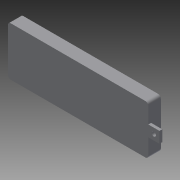
# Autodesk Inventor part: NodeMCU_holes
Saved by Autodesk Inventor 2014 SP1 (Build 180222100, 222)
## iProperties
Created: 2016-10-22
Part Number: NodeMCU_holes
Material: Generic
Document SubType Name: Modeling
Designer: danielsikar
Density: 1 g/cm^3
Appearance: Default
Author: danielsikar
Autodesk Inventor part; units mm, degrees
ref_plane "YZ Plane" through (0, 0, 0) normal (1, 0, 0) x (0, 1, 0)
ref_plane "XZ Plane" through (0, 0, 0) normal (0, 1, 0) x (-1, 0, 0)
ref_plane "XY Plane" through (0, 0, 0) normal (0, 0, 1) x (1, 0, 0)
sketch "Sketch1" plane through (0, 0, 0) normal (0, 1, 0) x (-1, 0, 0)
  line L0 (0, 0) -> (58, 0)
  line L1 (58, 0) -> (58, 31)
  line L2 (58, 31) -> (0, 31)
  circle A0 centre (3.1, 3.1) radius 1.6
  circle A1 centre (3.1, 27.9) radius 1.6
  circle A2 centre (54.9, 27.9) radius 1.6
  circle A3 centre (54.9, 3.1) radius 1.6
  circle A4 centre (-30.7, 7.25) radius 1.5
  circle A5 centre (-30.7, 23.75) radius 1.5
  line L3 (-38.5, 31) -> (-38.5, 0)
  line L4 (0, 31) -> (-38.5, 31)
  line L5 (0, 0) -> (-38.5, 0)
  line L6 (-38.5, 31) -> (58, 31)
  line L7 (58, 31) -> (58, 0)
  line L8 (58, 0) -> (-38.5, 0)
  line L9 (-38.5, 0) -> (-38.5, 31)
  circle A6 centre (-30.7, 23.75) radius 2.5
  circle A7 centre (-30.7, 7.25) radius 2.5
  circle A8 centre (3.1, 27.9) radius 2.5
  circle A9 centre (3.1, 3.1) radius 2.5
  circle A10 centre (54.9, 27.9) radius 2.5
  circle A11 centre (54.9, 3.1) radius 2.5
  dimension "d2" = 3.2
  dimension "d4" = 3.1
  dimension "d5" = 3.2
  dimension "d6" = 3.1
  dimension "d7" = 3.2
  dimension "d8" = 3.1
  dimension "d9" = 3.2
  dimension "d13" = 3
  dimension "d15" = 7.25
  dimension "d16" = 3
  dimension "d17" = 16.5
  dimension "d22" = 5
  dimension "d23" = 5
  dimension "d24" = 5
  dimension "d25" = 5
  dimension "d26" = 5
  dimension "d27" = 5
  constraints: 20 end point, 12 centre point, 6 coincident, 4 parallel, 3 perpendicular, 2 horizontal
  measures "d2" diameter of A0
  measures "d4" distance from line of A0.centre L0
  measures "d5" diameter of A1
  measures "d6" distance from line of A1.centre L2
  measures "d7" diameter of A2
  measures "d8" distance from line of L1 A2.centre
  measures "d9" diameter of A3
  measures "d13" diameter of A4
  measures "d15" distance from line of L0 A4.centre
  measures "d16" diameter of A5
  measures "d17" distance of A5.centre A4.centre
  measures "d22" diameter of A6
  measures "d23" diameter of A7
  measures "d24" diameter of A8
  measures "d25" diameter of A9
  measures "d26" diameter of A10
  measures "d27" diameter of A11
sketch "Sketch2" plane through (0, 0, 0) normal (0, 1, 0) x (-1, 0, 0)
  line L0 (-38.5, 31) -> (58, 31)
  line L1 (58, 31) -> (58, 0)
  line L2 (58, 0) -> (-38.5, 0)
  line L3 (-38.5, 0) -> (-38.5, 31)
  point P0 (0, 0)
  dimension "d19" = 96.5
  constraints: 8 end point, 2 parallel, 1 horizontal, 1 perpendicular
  measures "d19" distance of L1.end L2.end
extrude "Extrusion2" add sketch "Sketch2" along normal blind 2
extrude "Extrusion3" add sketch "Sketch1" along normal blind 9 contours A6 | A7 | A8 | A9 | A10 | A11
sketch "Sketch3" plane through (0, 0, 0) normal (0, -1, 0) x (1, 0, 0)
  line L0 (-58, 0) -> (38.5, 0) projected
  line L1 (38.5, 0) -> (38.5, 31) projected
  line L2 (-60, 33) -> (40.5, 33)
  line L3 (40.5, 33) -> (40.5, -2)
  line L4 (40.5, -2) -> (-60, -2)
  line L5 (-60, -2) -> (-60, 33)
  line L6 (-58, 31) -> (38.5, 31)
  line L7 (38.5, 31) -> (38.5, 0)
  line L8 (38.5, 0) -> (-58, 0)
  line L9 (-58, 0) -> (-58, 31)
  point P0 (0, 0)
  dimension "d30" = 35
  dimension "d31" = 100.5
  dimension "d32" = 2
  dimension "d33" = 2
  constraints: 16 end point, 4 parallel, 2 horizontal, 2 perpendicular
  measures "d30" distance between parallel lines of L4 L2
  measures "d31" distance between parallel lines of L5 L3
  measures "d32" distance between parallel lines of L1 L3
  measures "d33" distance between parallel lines of L4 L0
extrude "Extrusion4" add sketch "Sketch3" against normal blind 9
fillet "Fillet2" radius 2 4 edges at (-60, 4.5, -2) (40.5, 4.5, -2) (40.5, 4.5, 33) (-60, 4.5, 33)
sketch "Sketch5" plane through (40.5, 0, 31) normal (1, 0, 0) x (0, 0, -1)
  line L0 (0, 0) -> (31, 0) projected
  line L1 (11.5, 0) -> (19.5, 0)
  line L2 (19.5, 0) -> (19.5, 2)
  line L3 (19.5, 2) -> (11.5, 2)
  line L4 (11.5, 2) -> (11.5, 0)
  line L5 (-2, 9) -> (-2, 0) projected
  dimension "d37" = 8
  dimension "d38" = 2
  dimension "d39" = 13.5
  constraints: 8 end point, 2 parallel, 1 horizontal, 1 perpendicular, 1 point on line
  measures "d37" distance of L3.end L2.end
  measures "d38" distance of L2.end L1.end
  measures "d39" distance from line of L3.end L5
extrude "Extrusion5" add sketch "Sketch5" along normal blind 8
sketch "Sketch6" plane through (40.5, 2, 19.5) normal (0, 1, 0) x (1, 0, 0)
  circle A0 centre (4, 4) radius 1.5
  point P0 (-40.5, 19.5)
  dimension "d42" = 3
  constraints: 1 centre point
  measures "d42" diameter of A0
extrude "Extrusion6" cut sketch "Sketch6" against normal blind 2
fillet "Fillet7" radius 2 1 edges at (-9.75, 2, 0)
fillet "Fillet8" radius 2 4 edges at (38.5, 2.5858, 0.5858) (38.5, 6.5, 0) (38.5, 2, 16.5) (-9.75, 2, 31)
body "Solid2"
